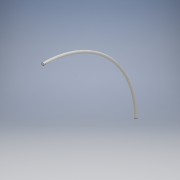
# Autodesk Inventor part: ArcRod
Saved by Autodesk Inventor 2018 (Build 220112000, 112)
## iProperties
Created: 2019-05-31
Part Number: ArcRod
Material: Generic
Document SubType Name: Modeling
Designer: ch1180245
Density: 1 g/cm^3
Appearance: Default
Author: ch1180245
Autodesk Inventor part; units mm, degrees
ref_plane "YZ Plane" through (0, 0, 0) normal (1, 0, 0) x (0, 1, 0)
ref_plane "XZ Plane" through (0, 0, 0) normal (0, 1, 0) x (-1, 0, 0)
ref_plane "XY Plane" through (0, 0, 0) normal (0, 0, 1) x (1, 0, 0)
sketch "Sketch2" plane through (0, 0, 0) normal (0, 0, 1) x (1, 0, 0)
  circle A0 centre (0, 750) radius 10
  point P0 (0, 0)
  dimension "d6" = 20
  dimension "d7" = 750
  constraints: 1 centre point
  measures "d6" diameter of A0
  measures "d7" distance of point (0, 0) A0.centre
sketch "Sketch3" plane through (0, 0, 0) normal (1, 0, 0) x (0, 1, 0)
  arc A0 (750, 0) -> (0, 750) centre (0, 0) ccw
  constraints: 2 point on circle, 1 centre point, 1 coincident
sweep "Sweep1" add profiles "Sketch2" path "Sketch3"
sketch "Sketch4" plane through (0, 0, 0) normal (1, 0, 0) x (0, 1, 0)
  circle A0 centre (12.9679, 750) radius 2.5
  point P0 (0, 0)
  dimension "d10" = 5
  constraints: 1 centre point
  measures "d10" diameter of A0
extrude "Extrusion1" cut sketch "Sketch4" along normal mid plane 60
body "Solid1"
